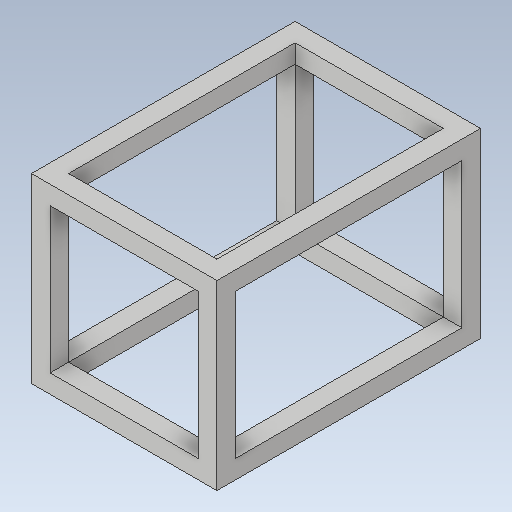
# Autodesk Inventor part: Motor Pump Housing
Saved by Autodesk Inventor 2020 (Build 240168000, 168)
## iProperties
Created: 2020-10-15
Part Number: Motor Pump Housing
Material: Generic
Document SubType Name: Modeling
Designer: nabee
Density: 1 g/cm^3
Appearance: Default
Author: nabee
Autodesk Inventor part; units mm, degrees
ref_plane "YZ Plane" through (0, 0, 0) normal (1, 0, 0) x (0, 1, 0)
ref_plane "XZ Plane" through (0, 0, 0) normal (0, 1, 0) x (-1, 0, 0)
ref_plane "XY Plane" through (0, 0, 0) normal (0, 0, 1) x (1, 0, 0)
sketch "Sketch1" plane through (0, 0, 0) normal (0, 0, 1) x (1, 0, 0)
  line L0 (0, 0) -> (200, 0)
  line L1 (200, 0) -> (200, 196.27)
  line L2 (200, 196.27) -> (0, 196.27)
  line L3 (0, 196.27) -> (0, 0)
  dimension "d0" = 200
  dimension "d1" = 196.27
  constraints: 8 end point, 2 parallel, 1 horizontal, 1 perpendicular
  measures "d0" distance of L2.end L1.end
  measures "d1" distance of L2.end L0.start
extrude "Extrusion1" add sketch "Sketch1" along normal blind 284.3
sketch "Sketch2" plane through (0, 0, 284.3) normal (0, 0, 1) x (1, 0, 0)
  line L0 (20, 176.27) -> (180, 176.27)
  line L1 (180, 176.27) -> (180, 20)
  line L2 (180, 20) -> (20, 20)
  line L3 (20, 20) -> (20, 176.27)
  line L4 (200, 196.27) -> (0, 196.27) projected
  line L5 (0, 196.27) -> (0, 0) projected
  line L6 (200, 0) -> (200, 196.27) projected
  line L7 (0, 0) -> (200, 0) projected
  dimension "d4" = 20
  dimension "d5" = 20
  dimension "d6" = 20
  dimension "d7" = 20
  constraints: 8 end point, 2 parallel, 1 horizontal, 1 perpendicular
  measures "d4" distance between parallel lines of L4 L0
  measures "d5" distance between parallel lines of L5 L3
  measures "d6" distance between parallel lines of L6 L1
  measures "d7" distance between parallel lines of L7 L2
extrude "Extrusion2" cut sketch "Sketch2" against normal blind 900 contours L0 L1 L2 L3
sketch "Sketch3" plane through (200, 0, 0) normal (1, 0, 0) x (0, 0, -1)
  line L0 (-264.3, 176.27) -> (-20, 176.27)
  line L1 (-20, 176.27) -> (-20, 20)
  line L2 (-20, 20) -> (-264.3, 20)
  line L3 (-264.3, 20) -> (-264.3, 176.27)
  line L4 (0, 196.27) -> (-284.3, 196.27) projected
  line L5 (-284.3, 0) -> (-284.3, 196.27) projected
  line L6 (0, 0) -> (-284.3, 0) projected
  line L7 (0, 0) -> (0, 196.27) projected
  dimension "d10" = 20
  dimension "d11" = 20
  dimension "d12" = 20
  dimension "d13" = 20
  constraints: 8 end point, 2 parallel, 1 horizontal, 1 perpendicular
  measures "d10" distance between parallel lines of L4 L0
  measures "d11" distance between parallel lines of L5 L3
  measures "d12" distance between parallel lines of L6 L2
  measures "d13" distance between parallel lines of L7 L1
extrude "Extrusion3" cut sketch "Sketch3" against normal blind 900 contours L0 L1 L2 L3
sketch "Sketch4" plane through (0, 196.27, 0) normal (0, 1, 0) x (1, 0, 0)
  line L0 (20, -264.3) -> (0, -264.3) projected
  line L1 (180, -20) -> (180, 0) projected
  line L2 (20, -264.3) -> (180, -264.3)
  line L3 (180, -264.3) -> (180, -20)
  line L4 (180, -20) -> (20, -20)
  line L5 (20, -20) -> (20, -264.3)
  point P0 (0, 0)
  constraints: 8 end point, 2 parallel, 1 horizontal, 1 perpendicular
extrude "Extrusion4" cut sketch "Sketch4" against normal blind 900
body "Solid1"
